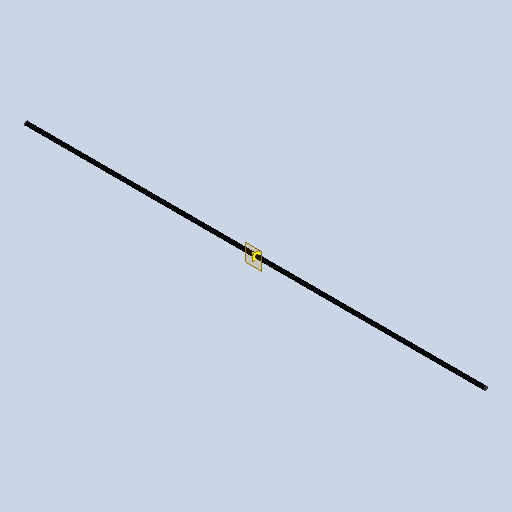
# Autodesk Inventor part: 6P-002
Saved by Autodesk Inventor 2025.2 (Build 292293000, 293)
## iProperties
Category: Main Assemply
Company: A
Created: 2024-10-31
Part Number: 6P-002
Material: CFRP
Document SubType Name: Modeling
Designer: Lachlan Uttley
Density: 1.43 g/cm^3
Appearance: Carbon Fiber
Mass: 5.78631 g
Surface Area: 81.4301 cm^2
Volume: 4.04637 cm^3
Title: HTP SPAR
Author: Lachlan Uttley
Revision Number: 1
Autodesk Inventor part; units mm, degrees
ref_plane "YZ Plane" through (0, 0, 0) normal (1, 0, 0) x (0, 1, 0)
ref_plane "XZ Plane" through (0, 0, 0) normal (0, 1, 0) x (-1, 0, 0)
ref_plane "XY Plane" through (0, 0, 0) normal (0, 0, 1) x (1, 0, 0)
sketch "Sketch7" plane through (0, 0, 0) normal (1, 0, 0) x (0, 1, 0)
  circle A0 centre (0, 0) radius 1.5
  circle A1 centre (0, 0) radius 2.5
  dimension "d85" = 3
  dimension "d86" = 5
  constraints: 3 coincident, 2 centre point
  measures "d85" diameter of A0
  measures "d86" diameter of A1
extrude "Extrusion3" add sketch "Sketch7" along normal blind 601
ref_plane "Work Plane2" through (300.5, 0, 0) normal (1, 0, 0) x (0, 0, -1)
sketch "Sketch8" plane through (300.5, 0, 0) normal (1, 0, 0) x (0, 0, -1)
  circle A0 centre (0, 0) radius 2.5 projected
  line L0 (-2.5, 0) -> (2.5, 0)
  constraints: 2 end point, 2 point on circle, 1 horizontal, 1 midpoint
ref_plane "Work Plane3" through (300.5, 0, 2.5) normal (0, 0, 1) x (1, 0, 0)
body "Solid2"
